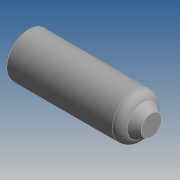
# Autodesk Inventor part: P110Poussoir
Saved by Autodesk Inventor 2015 SP1 (Build 190203100, 203)
## iProperties
Created: 2016-10-19
Part Number: P110Poussoir
Material: Générique
Document SubType Name: Modeling
Designer: serge.amoos
Density: 1 g/cm^3
Appearance: Par défaut
Author: serge.amoos
Autodesk Inventor part; units mm, degrees
ref_plane "YZ Plane" through (0, 0, 0) normal (1, 0, 0) x (0, 1, 0)
ref_plane "XZ Plane" through (0, 0, 0) normal (0, 1, 0) x (-1, 0, 0)
ref_plane "XY Plane" through (0, 0, 0) normal (0, 0, 1) x (1, 0, 0)
sketch "Sketch1" plane through (0, 0, 0) normal (0, 0, 1) x (1, 0, 0)
  line L0 (-16.8, 0) -> (2.8, 0) construction
  line L1 (0, -0.5) -> (0, 3) construction
  line L2 (0, 0) -> (0, 1.1726)
  line L3 (-1, 2.5) -> (-14, 2.5)
  line L4 (-14, 2.5) -> (-14, 1.75)
  line L5 (-14, 1.75) -> (-3, 1.75)
  line L6 (-3, 1.75) -> (-3, 0)
  line L7 (-3, 0) -> (0, 0)
  line L8 (-1, 2.5) -> (-1, 1.75)
  line L9 (-1, 1.75) -> (0, 1.1726)
  dimension "d0" = 5
  dimension "d1" = 3.5
  dimension "d3" = 14
  dimension "d6" = 2
  dimension "d7" = 60
  dimension "d9" = 1
  constraints: 16 end point, 3 perpendicular, 2 collinear, 2 point on line, 1 horizontal, 1 vertical
  measures "d0" diameter of L3 L0
  measures "d1" diameter of L5 L0
  measures "d3" distance between parallel lines of L1 L4
  measures "d6" distance between parallel lines of L8 L6
  measures "d7" angle of L1 L9
  measures "d9" distance between parallel lines of L1 L8
revolve "Revolution1" add sketch "Sketch1" angle 360 about axis through (-10, 0, 0) along (1, 0, 0)
fillet "Fillet2" radius 1 1 edges at (-1, -2.5, 0)
body "Solid1"
